Autodesk Fusion 360 part; units mm, degrees
(part 5 of 10)
  line L3608 (-26.7971, 36.5251) -> (-27.0734, 36.4711)
  line L3609 (-27.0734, 36.4711) -> (-27.3544, 36.4533)
  line L3610 (-27.3544, 36.4533) -> (-27.6353, 36.4722)
  line L3611 (-27.6353, 36.4722) -> (-27.9114, 36.5273)
  line L3612 (-27.9114, 36.5273) -> (-28.1781, 36.6178)
  line L3613 (-28.1781, 36.6178) -> (-28.4307, 36.7421)
  line L3614 (-28.4307, 36.7421) -> (-28.6651, 36.8981)
  line L3615 (-28.6651, 36.8981) -> (-28.8773, 37.0832)
  line L3616 (-28.8773, 37.0832) -> (-29.0637, 37.2942)
  line L3617 (-29.0637, 37.2942) -> (-29.2211, 37.5276)
  line L3618 (-29.2211, 37.5276) -> (-29.347, 37.7794)
  line L3619 (-29.347, 37.7794) -> (-29.4391, 38.0455)
  line L3620 (-29.4391, 38.0455) -> (-29.496, 38.3212)
  line L3621 (-29.496, 38.3212) -> (-29.5166, 38.602)
  line L3622 (-29.5166, 38.602) -> (-29.5006, 38.8831)
  line L3623 (-29.5006, 38.8831) -> (-29.4484, 39.1598)
  line L3624 (-29.4484, 39.1598) -> (-29.3606, 39.4273)
  line L3625 (-29.3606, 39.4273) -> (-29.3282, 39.495)
  line L3626 (-29.3282, 39.495) -> (-30.1357, 39.495)
  line L3627 (-30.1357, 39.495) -> (-30.1651, 39.411)
  line L3628 (-30.1651, 39.411) -> (-30.2382, 39.0907)
  line L3629 (-30.2382, 39.0907) -> (-30.275, 38.7643)
  line L3630 (-30.275, 38.7643) -> (-30.275, 38.4357)
  line L3631 (-26.8401, 42.0374) -> (-26.5056, 41.9709)
  line L3632 (-26.5056, 41.9709) -> (-26.1793, 41.8719)
  line L3633 (-26.1793, 41.8719) -> (-25.8642, 41.7414)
  line L3634 (-25.8642, 41.7414) -> (-25.5635, 41.5806)
  line L3635 (-25.5635, 41.5806) -> (-25.2799, 41.3911)
  line L3636 (-25.2799, 41.3911) -> (-25.0163, 41.1748)
  line L3637 (-25.0163, 41.1748) -> (-24.7752, 40.9337)
  line L3638 (-24.7752, 40.9337) -> (-24.5589, 40.6701)
  line L3639 (-24.5589, 40.6701) -> (-24.3694, 40.3865)
  line L3640 (-24.3694, 40.3865) -> (-24.2086, 40.0858)
  line L3641 (-24.2086, 40.0858) -> (-24.0781, 39.7707)
  line L3642 (-24.0781, 39.7707) -> (-23.9791, 39.4444)
  line L3643 (-23.9791, 39.4444) -> (-23.9126, 39.1099)
  line L3644 (-23.9126, 39.1099) -> (-23.8792, 38.7705)
  line L3645 (-23.8792, 38.7705) -> (-23.8792, 38.4295)
  line L3646 (-23.8792, 38.4295) -> (-23.9126, 38.0901)
  line L3647 (-23.9126, 38.0901) -> (-23.9791, 37.7556)
  line L3648 (-23.9791, 37.7556) -> (-24.0781, 37.4293)
  line L3649 (-24.0781, 37.4293) -> (-24.2086, 37.1142)
  line L3650 (-24.2086, 37.1142) -> (-24.3694, 36.8135)
  line L3651 (-24.3694, 36.8135) -> (-24.5589, 36.5299)
  line L3652 (-24.5589, 36.5299) -> (-24.7752, 36.2663)
  line L3653 (-24.7752, 36.2663) -> (-25.0163, 36.0252)
  line L3654 (-25.0163, 36.0252) -> (-25.2799, 35.8089)
  line L3655 (-25.2799, 35.8089) -> (-25.5635, 35.6194)
  line L3656 (-25.5635, 35.6194) -> (-25.8642, 35.4586)
  line L3657 (-25.8642, 35.4586) -> (-26.1793, 35.3281)
  line L3658 (-26.1793, 35.3281) -> (-26.5056, 35.2291)
  line L3659 (-26.5056, 35.2291) -> (-26.8401, 35.1626)
  line L3660 (-26.8401, 35.1626) -> (-27.1795, 35.1292)
  line L3661 (-27.1795, 35.1292) -> (-27.5205, 35.1292)
  line L3662 (-27.5205, 35.1292) -> (-27.8599, 35.1626)
  line L3663 (-27.8599, 35.1626) -> (-28.1944, 35.2291)
  line L3664 (-28.1944, 35.2291) -> (-28.5207, 35.3281)
  line L3665 (-28.5207, 35.3281) -> (-28.8358, 35.4586)
  line L3666 (-28.8358, 35.4586) -> (-29.1365, 35.6194)
  line L3667 (-29.1365, 35.6194) -> (-29.4201, 35.8089)
  line L3668 (-29.4201, 35.8089) -> (-29.6837, 36.0252)
  line L3669 (-29.6837, 36.0252) -> (-29.9248, 36.2663)
  line L3670 (-29.9248, 36.2663) -> (-30.1411, 36.5299)
  line L3671 (-30.1411, 36.5299) -> (-30.3306, 36.8135)
  line L3672 (-30.3306, 36.8135) -> (-30.4914, 37.1142)
  line L3673 (-30.4914, 37.1142) -> (-30.6219, 37.4293)
  line L3674 (-30.6219, 37.4293) -> (-30.7209, 37.7556)
  line L3675 (-30.7209, 37.7556) -> (-30.7874, 38.0901)
  line L3676 (-30.7874, 38.0901) -> (-30.8208, 38.4295)
  line L3677 (-30.8208, 38.4295) -> (-30.8208, 38.7705)
  line L3678 (-30.8208, 38.7705) -> (-30.8198, 38.7811)
  line L3679 (-30.8198, 38.7811) -> (-30.7874, 39.1099)
  line L3680 (-30.7874, 39.1099) -> (-30.7209, 39.4444)
  line L3681 (-30.7209, 39.4444) -> (-30.6219, 39.7707)
  line L3682 (-30.6219, 39.7707) -> (-30.4914, 40.0858)
  line L3683 (-30.4914, 40.0858) -> (-30.3306, 40.3865)
  line L3684 (-30.3306, 40.3865) -> (-30.1411, 40.6701)
  line L3685 (-30.1411, 40.6701) -> (-29.9248, 40.9337)
  line L3686 (-29.9248, 40.9337) -> (-29.6837, 41.1748)
  line L3687 (-29.6837, 41.1748) -> (-29.4201, 41.3911)
  line L3688 (-29.4201, 41.3911) -> (-29.1365, 41.5806)
  line L3689 (-29.1365, 41.5806) -> (-28.8358, 41.7414)
  line L3690 (-28.8358, 41.7414) -> (-28.5207, 41.8719)
  line L3691 (-28.5207, 41.8719) -> (-28.1944, 41.9709)
  line L3692 (-28.1944, 41.9709) -> (-27.8599, 42.0374)
  line L3693 (-27.8599, 42.0374) -> (-27.5205, 42.0708)
  line L3694 (-27.5205, 42.0708) -> (-27.1795, 42.0708)
  line L3695 (-27.1795, 42.0708) -> (-26.8401, 42.0374)
  line L3696 (-30.575, 38.4189) -> (-30.5344, 38.0589)
  line L3697 (-30.5344, 38.0589) -> (-30.4538, 37.7058)
  line L3698 (-30.4538, 37.7058) -> (-30.3342, 37.3639)
  line L3699 (-30.3342, 37.3639) -> (-30.177, 37.0375)
  line L3700 (-30.177, 37.0375) -> (-29.9843, 36.7308)
  line L3701 (-29.9843, 36.7308) -> (-29.7585, 36.4476)
  line L3702 (-29.7585, 36.4476) -> (-29.5024, 36.1915)
  line L3703 (-29.5024, 36.1915) -> (-29.2192, 35.9657)
  line L3704 (-29.2192, 35.9657) -> (-28.9125, 35.773)
  line L3705 (-28.9125, 35.773) -> (-28.5861, 35.6158)
  line L3706 (-28.5861, 35.6158) -> (-28.2442, 35.4962)
  line L3707 (-28.2442, 35.4962) -> (-27.8911, 35.4156)
  line L3708 (-27.8911, 35.4156) -> (-27.5311, 35.375)
  line L3709 (-27.5311, 35.375) -> (-27.1689, 35.375)
  line L3710 (-27.1689, 35.375) -> (-26.8089, 35.4156)
  line L3711 (-26.8089, 35.4156) -> (-26.4558, 35.4962)
  line L3712 (-26.4558, 35.4962) -> (-26.1139, 35.6158)
  line L3713 (-26.1139, 35.6158) -> (-25.7875, 35.773)
  line L3714 (-25.7875, 35.773) -> (-25.4808, 35.9657)
  line L3715 (-25.4808, 35.9657) -> (-25.1976, 36.1915)
  line L3716 (-25.1976, 36.1915) -> (-24.9415, 36.4476)
  line L3717 (-24.9415, 36.4476) -> (-24.7157, 36.7308)
  line L3718 (-24.7157, 36.7308) -> (-24.523, 37.0375)
  line L3719 (-24.523, 37.0375) -> (-24.3658, 37.3639)
  line L3720 (-24.3658, 37.3639) -> (-24.2462, 37.7058)
  line L3721 (-24.2462, 37.7058) -> (-24.1656, 38.0589)
  line L3722 (-24.1656, 38.0589) -> (-24.125, 38.4189)
  line L3723 (-24.125, 38.4189) -> (-24.125, 38.7811)
  line L3724 (-24.125, 38.7811) -> (-24.1656, 39.1411)
  line L3725 (-24.1656, 39.1411) -> (-24.2462, 39.4942)
  line L3726 (-24.2462, 39.4942) -> (-24.3658, 39.8361)
  line L3727 (-24.3658, 39.8361) -> (-24.523, 40.1625)
  line L3728 (-24.523, 40.1625) -> (-24.7157, 40.4692)
  line L3729 (-24.7157, 40.4692) -> (-24.9415, 40.7524)
  line L3730 (-24.9415, 40.7524) -> (-25.1976, 41.0085)
  line L3731 (-25.1976, 41.0085) -> (-25.4808, 41.2343)
  line L3732 (-25.4808, 41.2343) -> (-25.7875, 41.427)
  line L3733 (-25.7875, 41.427) -> (-26.1139, 41.5842)
  line L3734 (-26.1139, 41.5842) -> (-26.4558, 41.7038)
  line L3735 (-26.4558, 41.7038) -> (-26.8089, 41.7844)
  line L3736 (-26.8089, 41.7844) -> (-27.1689, 41.825)
  line L3737 (-27.1689, 41.825) -> (-27.5311, 41.825)
  line L3738 (-27.5311, 41.825) -> (-27.8911, 41.7844)
  line L3739 (-27.8911, 41.7844) -> (-28.2442, 41.7038)
  line L3740 (-28.2442, 41.7038) -> (-28.5861, 41.5842)
  line L3741 (-28.5861, 41.5842) -> (-28.9125, 41.427)
  line L3742 (-28.9125, 41.427) -> (-29.2192, 41.2343)
  line L3743 (-29.2192, 41.2343) -> (-29.5024, 41.0085)
  line L3744 (-29.5024, 41.0085) -> (-29.7585, 40.7524)
  line L3745 (-29.7585, 40.7524) -> (-29.9843, 40.4692)
  line L3746 (-29.9843, 40.4692) -> (-30.177, 40.1625)
  line L3747 (-30.177, 40.1625) -> (-30.3342, 39.8361)
  line L3748 (-30.3342, 39.8361) -> (-30.4538, 39.4942)
  line L3749 (-30.4538, 39.4942) -> (-30.5344, 39.1411)
  line L3750 (-30.5344, 39.1411) -> (-30.575, 38.7811)
  line L3751 (-30.575, 38.7811) -> (-30.575, 38.4189)
  line L3752 (-26.7535, 42.621) -> (-26.3623, 42.5432)
  line L3753 (-26.3623, 42.5432) -> (-25.9805, 42.4274)
  line L3754 (-25.9805, 42.4274) -> (-25.612, 42.2747)
  line L3755 (-25.612, 42.2747) -> (-25.2602, 42.0867)
  line L3756 (-25.2602, 42.0867) -> (-24.9285, 41.865)
  line L3757 (-24.9285, 41.865) -> (-24.6201, 41.612)
  line L3758 (-24.6201, 41.612) -> (-24.338, 41.3299)
  line L3759 (-24.338, 41.3299) -> (-24.085, 41.0215)
  line L3760 (-24.085, 41.0215) -> (-23.8633, 40.6898)
  line L3761 (-23.8633, 40.6898) -> (-23.6753, 40.338)
  line L3762 (-23.6753, 40.338) -> (-23.5226, 39.9695)
  line L3763 (-23.5226, 39.9695) -> (-23.4068, 39.5877)
  line L3764 (-23.4068, 39.5877) -> (-23.329, 39.1965)
  line L3765 (-23.329, 39.1965) -> (-23.2899, 38.7995)
  line L3766 (-23.2899, 38.7995) -> (-23.2899, 38.4005)
  line L3767 (-23.2899, 38.4005) -> (-23.329, 38.0035)
  line L3768 (-23.329, 38.0035) -> (-23.4068, 37.6123)
  line L3769 (-23.4068, 37.6123) -> (-23.5226, 37.2305)
  line L3770 (-23.5226, 37.2305) -> (-23.6753, 36.862)
  line L3771 (-23.6753, 36.862) -> (-23.8633, 36.5102)
  line L3772 (-23.8633, 36.5102) -> (-24.085, 36.1785)
  line L3773 (-24.085, 36.1785) -> (-24.338, 35.8701)
  line L3774 (-24.338, 35.8701) -> (-24.6201, 35.588)
  line L3775 (-24.6201, 35.588) -> (-24.9285, 35.335)
  line L3776 (-24.9285, 35.335) -> (-25.2602, 35.1133)
  line L3777 (-25.2602, 35.1133) -> (-25.612, 34.9253)
  line L3778 (-25.612, 34.9253) -> (-25.9805, 34.7726)
  line L3779 (-25.9805, 34.7726) -> (-26.3623, 34.6568)
  line L3780 (-26.3623, 34.6568) -> (-26.7535, 34.579)
  line L3781 (-26.7535, 34.579) -> (-27.1505, 34.5399)
  line L3782 (-27.1505, 34.5399) -> (-27.5495, 34.5399)
  line L3783 (-27.5495, 34.5399) -> (-27.9465, 34.579)
  line L3784 (-27.9465, 34.579) -> (-28.3377, 34.6568)
  line L3785 (-28.3377, 34.6568) -> (-28.7195, 34.7726)
  line L3786 (-28.7195, 34.7726) -> (-29.088, 34.9253)
  line L3787 (-29.088, 34.9253) -> (-29.4398, 35.1133)
  line L3788 (-29.4398, 35.1133) -> (-29.7715, 35.335)
  line L3789 (-29.7715, 35.335) -> (-30.0799, 35.588)
  line L3790 (-30.0799, 35.588) -> (-30.362, 35.8701)
  line L3791 (-30.362, 35.8701) -> (-30.615, 36.1785)
  line L3792 (-30.615, 36.1785) -> (-30.8367, 36.5102)
  line L3793 (-30.8367, 36.5102) -> (-31.0247, 36.862)
  line L3794 (-31.0247, 36.862) -> (-31.1774, 37.2305)
  line L3795 (-31.1774, 37.2305) -> (-31.2932, 37.6123)
  line L3796 (-31.2932, 37.6123) -> (-31.371, 38.0035)
  line L3797 (-31.371, 38.0035) -> (-31.4101, 38.4005)
  line L3798 (-31.4101, 38.4005) -> (-31.4101, 38.7874)
  line L3799 (-31.4101, 38.7874) -> (-31.4101, 38.7995)
  line L3800 (-31.4101, 38.7995) -> (-31.371, 39.1965)
  line L3801 (-31.371, 39.1965) -> (-31.2932, 39.5877)
  line L3802 (-31.2932, 39.5877) -> (-31.1774, 39.9695)
  line L3803 (-31.1774, 39.9695) -> (-31.0247, 40.338)
  line L3804 (-31.0247, 40.338) -> (-30.8367, 40.6898)
  line L3805 (-30.8367, 40.6898) -> (-30.615, 41.0215)
  line L3806 (-30.615, 41.0215) -> (-30.362, 41.3299)
  line L3807 (-30.362, 41.3299) -> (-30.0799, 41.612)
  line L3808 (-30.0799, 41.612) -> (-29.7715, 41.865)
  line L3809 (-29.7715, 41.865) -> (-29.4398, 42.0867)
  line L3810 (-29.4398, 42.0867) -> (-29.088, 42.2747)
  line L3811 (-29.088, 42.2747) -> (-28.7195, 42.4274)
  line L3812 (-28.7195, 42.4274) -> (-28.3377, 42.5432)
  line L3813 (-28.3377, 42.5432) -> (-27.9465, 42.621)
  line L3814 (-27.9465, 42.621) -> (-27.5495, 42.6601)
  line L3815 (-27.5495, 42.6601) -> (-27.1505, 42.6601)
  line L3816 (-27.1505, 42.6601) -> (-26.7535, 42.621)
  line L3817 (-31.165, 38.4126) -> (-31.1283, 38.0395)
  line L3818 (-31.1283, 38.0395) -> (-31.0551, 37.6719)
  line L3819 (-31.0551, 37.6719) -> (-30.9463, 37.3132)
  line L3820 (-30.9463, 37.3132) -> (-30.8029, 36.9669)
  line L3821 (-30.8029, 36.9669) -> (-30.6262, 36.6363)
  line L3822 (-30.6262, 36.6363) -> (-30.4179, 36.3247)
  line L3823 (-30.4179, 36.3247) -> (-30.1801, 36.0349)
  line L3824 (-30.1801, 36.0349) -> (-29.9151, 35.7699)
  line L3825 (-29.9151, 35.7699) -> (-29.6253, 35.5321)
  line L3826 (-29.6253, 35.5321) -> (-29.3137, 35.3238)
  line L3827 (-29.3137, 35.3238) -> (-28.9831, 35.1471)
  line L3828 (-28.9831, 35.1471) -> (-28.6368, 35.0037)
  line L3829 (-28.6368, 35.0037) -> (-28.2781, 34.8949)
  line L3830 (-28.2781, 34.8949) -> (-27.9105, 34.8217)
  line L3831 (-27.9105, 34.8217) -> (-27.5374, 34.785)
  line L3832 (-27.5374, 34.785) -> (-27.1626, 34.785)
  line L3833 (-27.1626, 34.785) -> (-26.7895, 34.8217)
  line L3834 (-26.7895, 34.8217) -> (-26.4219, 34.8949)
  line L3835 (-26.4219, 34.8949) -> (-26.0632, 35.0037)
  line L3836 (-26.0632, 35.0037) -> (-25.7169, 35.1471)
  line L3837 (-25.7169, 35.1471) -> (-25.3863, 35.3238)
  line L3838 (-25.3863, 35.3238) -> (-25.0747, 35.5321)
  line L3839 (-25.0747, 35.5321) -> (-24.7849, 35.7699)
  line L3840 (-24.7849, 35.7699) -> (-24.5199, 36.0349)
  line L3841 (-24.5199, 36.0349) -> (-24.2821, 36.3247)
  line L3842 (-24.2821, 36.3247) -> (-24.0738, 36.6363)
  line L3843 (-24.0738, 36.6363) -> (-23.8971, 36.9669)
  line L3844 (-23.8971, 36.9669) -> (-23.7537, 37.3132)
  line L3845 (-23.7537, 37.3132) -> (-23.6449, 37.6719)
  line L3846 (-23.6449, 37.6719) -> (-23.5717, 38.0395)
  line L3847 (-23.5717, 38.0395) -> (-23.535, 38.4126)
  line L3848 (-23.535, 38.4126) -> (-23.535, 38.7874)
  line L3849 (-23.535, 38.7874) -> (-23.5717, 39.1605)
  line L3850 (-23.5717, 39.1605) -> (-23.6449, 39.5281)
  line L3851 (-23.6449, 39.5281) -> (-23.7537, 39.8868)
  line L3852 (-23.7537, 39.8868) -> (-23.8971, 40.2331)
  line L3853 (-23.8971, 40.2331) -> (-24.0738, 40.5637)
  line L3854 (-24.0738, 40.5637) -> (-24.2821, 40.8753)
  line L3855 (-24.2821, 40.8753) -> (-24.5199, 41.1651)
  line L3856 (-24.5199, 41.1651) -> (-24.7849, 41.4301)
  line L3857 (-24.7849, 41.4301) -> (-25.0747, 41.6679)
  line L3858 (-25.0747, 41.6679) -> (-25.3863, 41.8762)
  line L3859 (-25.3863, 41.8762) -> (-25.7169, 42.0529)
  line L3860 (-25.7169, 42.0529) -> (-26.0632, 42.1963)
  line L3861 (-26.0632, 42.1963) -> (-26.4219, 42.3051)
  line L3862 (-26.4219, 42.3051) -> (-26.7895, 42.3783)
  line L3863 (-26.7895, 42.3783) -> (-27.1626, 42.415)
  line L3864 (-27.1626, 42.415) -> (-27.5374, 42.415)
  line L3865 (-27.5374, 42.415) -> (-27.9105, 42.3783)
  line L3866 (-27.9105, 42.3783) -> (-28.2781, 42.3051)
  line L3867 (-28.2781, 42.3051) -> (-28.6368, 42.1963)
  line L3868 (-28.6368, 42.1963) -> (-28.9831, 42.0529)
  line L3869 (-28.9831, 42.0529) -> (-29.3137, 41.8762)
  line L3870 (-29.3137, 41.8762) -> (-29.6253, 41.6679)
  line L3871 (-29.6253, 41.6679) -> (-29.9151, 41.4301)
  line L3872 (-29.9151, 41.4301) -> (-30.1801, 41.1651)
  line L3873 (-30.1801, 41.1651) -> (-30.4179, 40.8753)
  line L3874 (-30.4179, 40.8753) -> (-30.6262, 40.5637)
  line L3875 (-30.6262, 40.5637) -> (-30.8029, 40.2331)
  line L3876 (-30.8029, 40.2331) -> (-30.9463, 39.8868)
  line L3877 (-30.9463, 39.8868) -> (-31.0551, 39.5281)
  line L3878 (-31.0551, 39.5281) -> (-31.1283, 39.1605)
  line L3879 (-31.1283, 39.1605) -> (-31.165, 38.7874)
  line L3880 (-31.165, 38.7874) -> (-31.165, 38.4126)
  line L3881 (-30.3956, 44.7226) -> (-30.3506, 44.7039)
  line L3882 (-30.3506, 44.7039) -> (-30.3161, 44.6694)
  line L3883 (-30.3161, 44.6694) -> (-30.2974, 44.6244)
  line L3884 (-30.2974, 44.6244) -> (-30.2974, 44.5756)
  line L3885 (-30.2974, 44.5756) -> (-30.3161, 44.5306)
  line L3886 (-30.3161, 44.5306) -> (-30.3506, 44.4961)
  line L3887 (-30.3506, 44.4961) -> (-30.3956, 44.4774)
  line L3888 (-30.3956, 44.4774) -> (-30.42, 44.475)
  line L3889 (-30.42, 44.475) -> (-33.04, 44.475)
  line L3890 (-33.04, 44.475) -> (-33.0644, 44.4774)
  line L3891 (-33.0644, 44.4774) -> (-33.1094, 44.4961)
  line L3892 (-33.1094, 44.4961) -> (-33.125, 44.5116)
  line L3893 (-33.125, 44.5116) -> (-33.125, 40.77)
  line L3894 (-33.125, 40.77) -> (-33.1274, 40.7456)
  line L3895 (-33.1274, 40.7456) -> (-33.1461, 40.7006)
  line L3896 (-33.1461, 40.7006) -> (-33.1806, 40.6661)
  line L3897 (-33.1806, 40.6661) -> (-33.2256, 40.6474)
  line L3898 (-33.2256, 40.6474) -> (-33.2744, 40.6474)
  line L3899 (-33.2744, 40.6474) -> (-33.3194, 40.6661)
  line L3900 (-33.3194, 40.6661) -> (-33.3539, 40.7006)
  line L3901 (-33.3539, 40.7006) -> (-33.3726, 40.7456)
  line L3902 (-33.3726, 40.7456) -> (-33.375, 40.77)
  line L3903 (-33.375, 40.77) -> (-33.375, 44.6)
  line L3904 (-33.375, 44.6) -> (-33.3726, 44.6244)
  line L3905 (-33.3726, 44.6244) -> (-33.3539, 44.6694)
  line L3906 (-33.3539, 44.6694) -> (-33.3194, 44.7039)
  line L3907 (-33.3194, 44.7039) -> (-33.2744, 44.7226)
  line L3908 (-33.2744, 44.7226) -> (-33.2256, 44.7226)
  line L3909 (-33.2256, 44.7226) -> (-33.1806, 44.7039)
  line L3910 (-33.1806, 44.7039) -> (-33.1461, 44.6694)
  line L3911 (-33.1461, 44.6694) -> (-33.145, 44.6669)
  line L3912 (-33.145, 44.6669) -> (-33.1439, 44.6694)
  line L3913 (-33.1439, 44.6694) -> (-33.1094, 44.7039)
  line L3914 (-33.1094, 44.7039) -> (-33.0644, 44.7226)
  line L3915 (-33.0644, 44.7226) -> (-33.04, 44.725)
  line L3916 (-33.04, 44.725) -> (-30.42, 44.725)
  line L3917 (-30.42, 44.725) -> (-30.3956, 44.7226)
  line L3918 (-21.4256, 44.7226) -> (-21.3806, 44.7039)
  line L3919 (-21.3806, 44.7039) -> (-21.3461, 44.6694)
  line L3920 (-21.3461, 44.6694) -> (-21.3274, 44.6244)
  line L3921 (-21.3274, 44.6244) -> (-21.325, 44.6)
  line L3922 (-21.325, 44.6) -> (-21.325, 40.77)
  line L3923 (-21.325, 40.77) -> (-21.3274, 40.7456)
  line L3924 (-21.3274, 40.7456) -> (-21.3461, 40.7006)
  line L3925 (-21.3461, 40.7006) -> (-21.3806, 40.6661)
  line L3926 (-21.3806, 40.6661) -> (-21.4256, 40.6474)
  line L3927 (-21.4256, 40.6474) -> (-21.4744, 40.6474)
  line L3928 (-21.4744, 40.6474) -> (-21.5194, 40.6661)
  line L3929 (-21.5194, 40.6661) -> (-21.5539, 40.7006)
  line L3930 (-21.5539, 40.7006) -> (-21.5726, 40.7456)
  line L3931 (-21.5726, 40.7456) -> (-21.575, 40.77)
  line L3932 (-21.575, 40.77) -> (-21.575, 44.475)
  line L3933 (-21.575, 44.475) -> (-24.28, 44.475)
  line L3934 (-24.28, 44.475) -> (-24.3044, 44.4774)
  line L3935 (-24.3044, 44.4774) -> (-24.3494, 44.4961)
  line L3936 (-24.3494, 44.4961) -> (-24.3839, 44.5306)
  line L3937 (-24.3839, 44.5306) -> (-24.4026, 44.5756)
  line L3938 (-24.4026, 44.5756) -> (-24.4026, 44.6244)
  line L3939 (-24.4026, 44.6244) -> (-24.3839, 44.6694)
  line L3940 (-24.3839, 44.6694) -> (-24.3494, 44.7039)
  line L3941 (-24.3494, 44.7039) -> (-24.3044, 44.7226)
  line L3942 (-24.3044, 44.7226) -> (-24.28, 44.725)
  line L3943 (-24.28, 44.725) -> (-21.45, 44.725)
  line L3944 (-21.45, 44.725) -> (-21.4256, 44.7226)
  line L3945 (-25.3156, 44.7226) -> (-25.2706, 44.7039)
  line L3946 (-25.2706, 44.7039) -> (-25.2361, 44.6694)
  line L3947 (-25.2361, 44.6694) -> (-25.2174, 44.6244)
  line L3948 (-25.2174, 44.6244) -> (-25.2174, 44.5756)
  line L3949 (-25.2174, 44.5756) -> (-25.2361, 44.5306)
  line L3950 (-25.2361, 44.5306) -> (-25.2706, 44.4961)
  line L3951 (-25.2706, 44.4961) -> (-25.3156, 44.4774)
  line L3952 (-25.3156, 44.4774) -> (-25.34, 44.475)
  line L3953 (-25.34, 44.475) -> (-29.36, 44.475)
  line L3954 (-29.36, 44.475) -> (-29.3844, 44.4774)
  line L3955 (-29.3844, 44.4774) -> (-29.4294, 44.4961)
  line L3956 (-29.4294, 44.4961) -> (-29.4639, 44.5306)
  line L3957 (-29.4639, 44.5306) -> (-29.4826, 44.5756)
  line L3958 (-29.4826, 44.5756) -> (-29.4826, 44.6244)
  line L3959 (-29.4826, 44.6244) -> (-29.4639, 44.6694)
  line L3960 (-29.4639, 44.6694) -> (-29.4294, 44.7039)
  line L3961 (-29.4294, 44.7039) -> (-29.3844, 44.7226)
  line L3962 (-29.3844, 44.7226) -> (-29.36, 44.725)
  line L3963 (-29.36, 44.725) -> (-25.34, 44.725)
  line L3964 (-25.34, 44.725) -> (-25.3156, 44.7226)
  line L3965 (-21.4446, 45.773) -> (-21.4446, 45.727)
  line L3966 (-21.4446, 45.727) -> (-21.477, 45.6946)
  line L3967 (-21.477, 45.6946) -> (-21.523, 45.6946)
  line L3968 (-21.523, 45.6946) -> (-21.5554, 45.727)
  line L3969 (-21.5554, 45.727) -> (-21.5554, 45.773)
  line L3970 (-21.5554, 45.773) -> (-21.523, 45.8054)
  line L3971 (-21.523, 45.8054) -> (-21.477, 45.8054)
  line L3972 (-21.477, 45.8054) -> (-21.4446, 45.773)
  line L3973 (-15.9694, 47.7992) -> (-15.8993, 47.7291)
  line L3974 (-15.8993, 47.7291) -> (-15.8614, 47.6375)
  line L3975 (-15.8614, 47.6375) -> (-15.8614, 47.5384)
  line L3976 (-15.8614, 47.5384) -> (-15.8993, 47.4469)
  line L3977 (-15.8993, 47.4469) -> (-15.9694, 47.3768)
  line L3978 (-15.9694, 47.3768) -> (-16.0609, 47.3389)
  line L3979 (-16.0609, 47.3389) -> (-16.1601, 47.3389)
  line L3980 (-16.1601, 47.3389) -> (-16.2516, 47.3768)
  line L3981 (-16.2516, 47.3768) -> (-16.3217, 47.4469)
  line L3982 (-16.3217, 47.4469) -> (-16.3596, 47.5384)
  line L3983 (-16.3596, 47.5384) -> (-16.3596, 47.6375)
  line L3984 (-16.3596, 47.6375) -> (-16.3217, 47.7291)
  line L3985 (-16.3217, 47.7291) -> (-16.2516, 47.7992)
  line L3986 (-16.2516, 47.7992) -> (-16.1601, 47.8371)
  line L3987 (-16.1601, 47.8371) -> (-16.0609, 47.8371)
  line L3988 (-16.0609, 47.8371) -> (-15.9694, 47.7992)
  line L3989 (-27.5973, 48.6187) -> (-27.5948, 48.6177)
  line L3990 (-27.5948, 48.6177) -> (-27.5921, 48.6175)
  line L3991 (-27.5921, 48.6175) -> (-27.5784, 48.6123)
  line L3992 (-27.5784, 48.6123) -> (-27.4831, 48.5646)
  line L3993 (-27.4831, 48.5646) -> (-27.4768, 48.5607)
  line L3994 (-27.4768, 48.5607) -> (-27.475, 48.5599)
  line L3995 (-27.475, 48.5599) -> (-27.4729, 48.5582)
  line L3996 (-27.4729, 48.5582) -> (-27.4707, 48.5568)
  line L3997 (-27.4707, 48.5568) -> (-27.4694, 48.5553)
  line L3998 (-27.4694, 48.5553) -> (-27.4636, 48.5506)
  line L3999 (-27.4636, 48.5506) -> (-27.3684, 48.4554)
  line L4000 (-27.3684, 48.4554) -> (-27.3591, 48.444)
  line L4001 (-27.3591, 48.444) -> (-27.3569, 48.4388)
  line L4002 (-27.3569, 48.4388) -> (-27.3536, 48.4344)
  line L4003 (-27.3536, 48.4344) -> (-27.3487, 48.4205)
  line L4004 (-27.3487, 48.4205) -> (-27.301, 48.23)
  line L4005 (-27.301, 48.23) -> (-27.3007, 48.2275)
  line L4006 (-27.3007, 48.2275) -> (-27.3003, 48.2265)
  line L4007 (-27.3003, 48.2265) -> (-27.2997, 48.221)
  line L4008 (-27.2997, 48.221) -> (-27.2989, 48.2155)
  line L4009 (-27.2989, 48.2155) -> (-27.2991, 48.2144)
  line L4010 (-27.2991, 48.2144) -> (-27.2988, 48.2118)
  line L4011 (-27.2988, 48.2118) -> (-27.2988, 47.8785)
  line L4012 (-27.2988, 47.8785) -> (-27.2991, 47.876)
  line L4013 (-27.2991, 47.876) -> (-27.2989, 47.8749)
  line L4014 (-27.2989, 47.8749) -> (-27.2997, 47.8694)
  line L4015 (-27.2997, 47.8694) -> (-27.3003, 47.8639)
  line L4016 (-27.3003, 47.8639) -> (-27.3007, 47.8629)
  line L4017 (-27.3007, 47.8629) -> (-27.301, 47.8603)
  line L4018 (-27.301, 47.8603) -> (-27.3487, 47.6698)
  line L4019 (-27.3487, 47.6698) -> (-27.3536, 47.656)
  line L4020 (-27.3536, 47.656) -> (-27.3569, 47.6515)
  line L4021 (-27.3569, 47.6515) -> (-27.3591, 47.6464)
  line L4022 (-27.3591, 47.6464) -> (-27.3684, 47.635)
  line L4023 (-27.3684, 47.635) -> (-27.4636, 47.5398)
  line L4024 (-27.4636, 47.5398) -> (-27.4694, 47.535)
  line L4025 (-27.4694, 47.535) -> (-27.4707, 47.5335)
  line L4026 (-27.4707, 47.5335) -> (-27.4729, 47.5321)
  line L4027 (-27.4729, 47.5321) -> (-27.475, 47.5304)
  line L4028 (-27.475, 47.5304) -> (-27.4768, 47.5297)
  line L4029 (-27.4768, 47.5297) -> (-27.4831, 47.5257)
  line L4030 (-27.4831, 47.5257) -> (-27.5784, 47.4781)
  line L4031 (-27.5784, 47.4781) -> (-27.5921, 47.4728)
  line L4032 (-27.5921, 47.4728) -> (-27.5948, 47.4727)
  line L4033 (-27.5948, 47.4727) -> (-27.5973, 47.4716)
  line L4034 (-27.5973, 47.4716) -> (-27.6119, 47.4702)
  line L4035 (-27.6119, 47.4702) -> (-27.8024, 47.4702)
  line L4036 (-27.8024, 47.4702) -> (-27.817, 47.4716)
  line L4037 (-27.817, 47.4716) -> (-27.8195, 47.4727)
  line L4038 (-27.8195, 47.4727) -> (-27.8222, 47.4728)
  line L4039 (-27.8222, 47.4728) -> (-27.8359, 47.4781)
  line L4040 (-27.8359, 47.4781) -> (-27.9312, 47.5257)
  line L4041 (-27.9312, 47.5257) -> (-27.9375, 47.5297)
  line L4042 (-27.9375, 47.5297) -> (-27.9393, 47.5304)
  line L4043 (-27.9393, 47.5304) -> (-27.9413, 47.5321)
  line L4044 (-27.9413, 47.5321) -> (-27.9436, 47.5335)
  line L4045 (-27.9436, 47.5335) -> (-27.9449, 47.535)
  line L4046 (-27.9449, 47.535) -> (-27.9507, 47.5398)
  line L4047 (-27.9507, 47.5398) -> (-28.0459, 47.635)
  line L4048 (-28.0459, 47.635) -> (-28.0552, 47.6464)
  line L4049 (-28.0552, 47.6464) -> (-28.0574, 47.6515)
  line L4050 (-28.0574, 47.6515) -> (-28.0607, 47.656)
  line L4051 (-28.0607, 47.656) -> (-28.0656, 47.6698)
  line L4052 (-28.0656, 47.6698) -> (-28.1132, 47.8603)
  line L4053 (-28.1132, 47.8603) -> (-28.1136, 47.8629)
  line L4054 (-28.1136, 47.8629) -> (-28.114, 47.8639)
  line L4055 (-28.114, 47.8639) -> (-28.1146, 47.8694)
  line L4056 (-28.1146, 47.8694) -> (-28.1154, 47.8749)
  line L4057 (-28.1154, 47.8749) -> (-28.1152, 47.876)
  line L4058 (-28.1152, 47.876) -> (-28.1155, 47.8785)
  line L4059 (-28.1155, 47.8785) -> (-28.1155, 48.2118)
  line L4060 (-28.1155, 48.2118) -> (-28.1152, 48.2144)
  line L4061 (-28.1152, 48.2144) -> (-28.1154, 48.2155)
  line L4062 (-28.1154, 48.2155) -> (-28.1146, 48.221)
  line L4063 (-28.1146, 48.221) -> (-28.114, 48.2265)
  line L4064 (-28.114, 48.2265) -> (-28.1136, 48.2275)
  line L4065 (-28.1136, 48.2275) -> (-28.1132, 48.23)
  line L4066 (-28.1132, 48.23) -> (-28.0656, 48.4205)
  line L4067 (-28.0656, 48.4205) -> (-28.0607, 48.4344)
  line L4068 (-28.0607, 48.4344) -> (-28.0574, 48.4388)
  line L4069 (-28.0574, 48.4388) -> (-28.0552, 48.444)
  line L4070 (-28.0552, 48.444) -> (-28.0459, 48.4554)
  line L4071 (-28.0459, 48.4554) -> (-27.9507, 48.5506)
  line L4072 (-27.9507, 48.5506) -> (-27.9449, 48.5553)
  line L4073 (-27.9449, 48.5553) -> (-27.9436, 48.5568)
  line L4074 (-27.9436, 48.5568) -> (-27.9413, 48.5582)
  line L4075 (-27.9413, 48.5582) -> (-27.9393, 48.5599)
  line L4076 (-27.9393, 48.5599) -> (-27.9375, 48.5607)
  line L4077 (-27.9375, 48.5607) -> (-27.9312, 48.5646)
  line L4078 (-27.9312, 48.5646) -> (-27.8359, 48.6123)
  line L4079 (-27.8359, 48.6123) -> (-27.8222, 48.6175)
  line L4080 (-27.8222, 48.6175) -> (-27.8195, 48.6177)
  line L4081 (-27.8195, 48.6177) -> (-27.817, 48.6187)
  line L4082 (-27.817, 48.6187) -> (-27.8024, 48.6202)
  line L4083 (-27.8024, 48.6202) -> (-27.6119, 48.6202)
  line L4084 (-27.6119, 48.6202) -> (-27.5973, 48.6187)
  line L4085 (-27.8532, 48.4359) -> (-27.9251, 48.364)
  line L4086 (-27.9251, 48.364) -> (-27.9655, 48.2026)
  line L4087 (-27.9655, 48.2026) -> (-27.9655, 47.8877)
  line L4088 (-27.9655, 47.8877) -> (-27.9251, 47.7264)
  line L4089 (-27.9251, 47.7264) -> (-27.8532, 47.6544)
  line L4090 (-27.8532, 47.6544) -> (-27.7847, 47.6202)
  line L4091 (-27.7847, 47.6202) -> (-27.6296, 47.6202)
  line L4092 (-27.6296, 47.6202) -> (-27.5611, 47.6544)
  line L4093 (-27.5611, 47.6544) -> (-27.4892, 47.7264)
  line L4094 (-27.4892, 47.7264) -> (-27.4488, 47.8877)
  line L4095 (-27.4488, 47.8877) -> (-27.4488, 48.2026)
  line L4096 (-27.4488, 48.2026) -> (-27.4892, 48.364)
  line L4097 (-27.4892, 48.364) -> (-27.5611, 48.4359)
  line L4098 (-27.5611, 48.4359) -> (-27.6296, 48.4702)
  line L4099 (-27.6296, 48.4702) -> (-27.7847, 48.4702)
  line L4100 (-27.7847, 48.4702) -> (-27.8532, 48.4359)
  line L4101 (-25.938, 48.6187) -> (-25.9306, 48.6187)
  line L4102 (-25.9306, 48.6187) -> (-25.9238, 48.6159)
  line L4103 (-25.9238, 48.6159) -> (-25.9166, 48.6145)
  line L4104 (-25.9166, 48.6145) -> (-25.9104, 48.6104)
  line L4105 (-25.9104, 48.6104) -> (-25.9036, 48.6075)
  line L4106 (-25.9036, 48.6075) -> (-25.8984, 48.6023)
  line L4107 (-25.8984, 48.6023) -> (-25.8923, 48.5983)
  line L4108 (-25.8923, 48.5983) -> (-25.8881, 48.5921)
  line L4109 (-25.8881, 48.5921) -> (-25.8829, 48.5868)
  line L4110 (-25.8829, 48.5868) -> (-25.8801, 48.5801)
  line L4111 (-25.8801, 48.5801) -> (-25.876, 48.574)
  line L4112 (-25.876, 48.574) -> (-25.8745, 48.5667)
  line L4113 (-25.8745, 48.5667) -> (-25.8717, 48.5598)
  line L4114 (-25.8717, 48.5598) -> (-25.8703, 48.5453)
  line L4115 (-25.8703, 48.5453) -> (-25.8702, 48.5453)
  line L4116 (-25.8702, 48.5453) -> (-25.8702, 48.5452)
  line L4117 (-25.8702, 48.5452) -> (-25.8702, 48.5452)
  line L4118 (-25.8702, 48.5452) -> (-25.8702, 47.6202)
  line L4119 (-25.8702, 47.6202) -> (-25.6595, 47.6202)
  line L4120 (-25.6595, 47.6202) -> (-25.6449, 47.6187)
  line L4121 (-25.6449, 47.6187) -> (-25.6179, 47.6075)
  line L4122 (-25.6179, 47.6075) -> (-25.5972, 47.5868)
  line L4123 (-25.5972, 47.5868) -> (-25.586, 47.5598)
  line L4124 (-25.586, 47.5598) -> (-25.586, 47.5305)
  line L4125 (-25.586, 47.5305) -> (-25.5972, 47.5035)
  line L4126 (-25.5972, 47.5035) -> (-25.6179, 47.4828)
  line L4127 (-25.6179, 47.4828) -> (-25.6449, 47.4716)
  line L4128 (-25.6449, 47.4716) -> (-25.6595, 47.4702)
  line L4129 (-25.6595, 47.4702) -> (-26.231, 47.4702)
  line L4130 (-26.231, 47.4702) -> (-26.2456, 47.4716)
  line L4131 (-26.2456, 47.4716) -> (-26.2726, 47.4828)
  line L4132 (-26.2726, 47.4828) -> (-26.2933, 47.5035)
  line L4133 (-26.2933, 47.5035) -> (-26.3045, 47.5305)
  line L4134 (-26.3045, 47.5305) -> (-26.3045, 47.5598)
  line L4135 (-26.3045, 47.5598) -> (-26.2933, 47.5868)
  line L4136 (-26.2933, 47.5868) -> (-26.2726, 47.6075)
  line L4137 (-26.2726, 47.6075) -> (-26.2456, 47.6187)
  line L4138 (-26.2456, 47.6187) -> (-26.231, 47.6202)
  line L4139 (-26.231, 47.6202) -> (-26.0202, 47.6202)
  line L4140 (-26.0202, 47.6202) -> (-26.0202, 48.3165)
  line L4141 (-26.0202, 48.3165) -> (-26.0827, 48.2541)
  line L4142 (-26.0827, 48.2541) -> (-26.0884, 48.2493)
  line L4143 (-26.0884, 48.2493) -> (-26.0897, 48.2478)
  line L4144 (-26.0897, 48.2478) -> (-26.092, 48.2464)
  line L4145 (-26.092, 48.2464) -> (-26.094, 48.2447)
  line L4146 (-26.094, 48.2447) -> (-26.0959, 48.244)
  line L4147 (-26.0959, 48.244) -> (-26.1022, 48.24)
  line L4148 (-26.1022, 48.24) -> (-26.1974, 48.1924)
  line L4149 (-26.1974, 48.1924) -> (-26.2111, 48.1871)
  line L4150 (-26.2111, 48.1871) -> (-26.2403, 48.1851)
  line L4151 (-26.2403, 48.1851) -> (-26.2681, 48.1943)
  line L4152 (-26.2681, 48.1943) -> (-26.2902, 48.2135)
  line L4153 (-26.2902, 48.2135) -> (-26.3033, 48.2397)
  line L4154 (-26.3033, 48.2397) -> (-26.3054, 48.2688)
  line L4155 (-26.3054, 48.2688) -> (-26.2961, 48.2966)
  line L4156 (-26.2961, 48.2966) -> (-26.2769, 48.3187)
  line L4157 (-26.2769, 48.3187) -> (-26.2645, 48.3265)
  line L4158 (-26.2645, 48.3265) -> (-26.1801, 48.3687)
  line L4159 (-26.1801, 48.3687) -> (-26.0988, 48.4501)
  line L4160 (-26.0988, 48.4501) -> (-26.0076, 48.5868)
  line L4161 (-26.0076, 48.5868) -> (-26.0076, 48.5868)
  line L4162 (-26.0076, 48.5868) -> (-26.0076, 48.5868)
  line L4163 (-26.0076, 48.5868) -> (-26.0075, 48.5869)
  line L4164 (-26.0075, 48.5869) -> (-25.9983, 48.5982)
  line L4165 (-25.9983, 48.5982) -> (-25.9922, 48.6023)
  line L4166 (-25.9922, 48.6023) -> (-25.9869, 48.6075)
  line L4167 (-25.9869, 48.6075) -> (-25.9801, 48.6104)
  line L4168 (-25.9801, 48.6104) -> (-25.974, 48.6144)
  line L4169 (-25.974, 48.6144) -> (-25.9667, 48.6159)
  line L4170 (-25.9667, 48.6159) -> (-25.9599, 48.6187)
  line L4171 (-25.9599, 48.6187) -> (-25.9525, 48.6187)
  line L4172 (-25.9525, 48.6187) -> (-25.9453, 48.6202)
  line L4173 (-25.9453, 48.6202) -> (-25.938, 48.6187)
  line L4174 (-28.5973, 48.6187) -> (-28.5948, 48.6177)
  line L4175 (-28.5948, 48.6177) -> (-28.5921, 48.6175)
  line L4176 (-28.5921, 48.6175) -> (-28.5784, 48.6123)
  line L4177 (-28.5784, 48.6123) -> (-28.4831, 48.5646)
  line L4178 (-28.4831, 48.5646) -> (-28.4768, 48.5607)
  line L4179 (-28.4768, 48.5607) -> (-28.475, 48.5599)
  line L4180 (-28.475, 48.5599) -> (-28.4729, 48.5582)
  line L4181 (-28.4729, 48.5582) -> (-28.4707, 48.5568)
  line L4182 (-28.4707, 48.5568) -> (-28.4694, 48.5553)
  line L4183 (-28.4694, 48.5553) -> (-28.4636, 48.5506)
  line L4184 (-28.4636, 48.5506) -> (-28.416, 48.503)
  line L4185 (-28.416, 48.503) -> (-28.4113, 48.4972)
  line L4186 (-28.4113, 48.4972) -> (-28.4098, 48.4959)
  line L4187 (-28.4098, 48.4959) -> (-28.4084, 48.4937)
  line L4188 (-28.4084, 48.4937) -> (-28.4067, 48.4916)
  line L4189 (-28.4067, 48.4916) -> (-28.4059, 48.4898)
  line L4190 (-28.4059, 48.4898) -> (-28.402, 48.4835)
  line L4191 (-28.402, 48.4835) -> (-28.3543, 48.3882)
  line L4192 (-28.3543, 48.3882) -> (-28.3491, 48.3745)
  line L4193 (-28.3491, 48.3745) -> (-28.3489, 48.3718)
  line L4194 (-28.3489, 48.3718) -> (-28.3479, 48.3693)
  line L4195 (-28.3479, 48.3693) -> (-28.3464, 48.3547)
  line L4196 (-28.3464, 48.3547) -> (-28.3464, 48.2118)
  line L4197 (-28.3464, 48.2118) -> (-28.3479, 48.1972)
  line L4198 (-28.3479, 48.1972) -> (-28.3489, 48.1947)
  line L4199 (-28.3489, 48.1947) -> (-28.3491, 48.192)
  line L4200 (-28.3491, 48.192) -> (-28.3543, 48.1783)
  line L4201 (-28.3543, 48.1783) -> (-28.402, 48.0831)
  line L4202 (-28.402, 48.0831) -> (-28.4059, 48.0768)
  line L4203 (-28.4059, 48.0768) -> (-28.4067, 48.0749)
  line L4204 (-28.4067, 48.0749) -> (-28.4084, 48.0729)
  line L4205 (-28.4084, 48.0729) -> (-28.4098, 48.0706)
  line L4206 (-28.4098, 48.0706) -> (-28.4113, 48.0693)
  line L4207 (-28.4113, 48.0693) -> (-28.416, 48.0636)
  line L4208 (-28.416, 48.0636) -> (-28.4636, 48.016)
  line L4209 (-28.4636, 48.016) -> (-28.4694, 48.0112)
  line L4210 (-28.4694, 48.0112) -> (-28.4707, 48.0097)
  line L4211 (-28.4707, 48.0097) -> (-28.4729, 48.0083)
  line L4212 (-28.4729, 48.0083) -> (-28.475, 48.0066)
  line L4213 (-28.475, 48.0066) -> (-28.4768, 48.0059)
  line L4214 (-28.4768, 48.0059) -> (-28.4831, 48.0019)
  line L4215 (-28.4831, 48.0019) -> (-28.5784, 47.9543)
  line L4216 (-28.5784, 47.9543) -> (-28.5921, 47.949)
  line L4217 (-28.5921, 47.949) -> (-28.5948, 47.9488)
  line L4218 (-28.5948, 47.9488) -> (-28.5973, 47.9478)
  line L4219 (-28.5973, 47.9478) -> (-28.6108, 47.9465)
  line L4220 (-28.6108, 47.9465) -> (-28.36, 47.5882)
  line L4221 (-28.36, 47.5882) -> (-28.3528, 47.5754)
  line L4222 (-28.3528, 47.5754) -> (-28.3464, 47.5468)
  line L4223 (-28.3464, 47.5468) -> (-28.3515, 47.518)
  line L4224 (-28.3515, 47.518) -> (-28.3673, 47.4933)
  line L4225 (-28.3673, 47.4933) -> (-28.3912, 47.4765)
  line L4226 (-28.3912, 47.4765) -> (-28.4198, 47.4702)
  line L4227 (-28.4198, 47.4702) -> (-28.4486, 47.4753)
  line L4228 (-28.4486, 47.4753) -> (-28.4733, 47.491)
  line L4229 (-28.4733, 47.491) -> (-28.4829, 47.5022)
  line L4230 (-28.4829, 47.5022) -> (-28.7938, 47.9464)
  line L4231 (-28.7938, 47.9464) -> (-28.9179, 47.9464)
  line L4232 (-28.9179, 47.9464) -> (-28.9179, 47.5452)
  line L4233 (-28.9179, 47.5452) -> (-28.9193, 47.5305)
  line L4234 (-28.9193, 47.5305) -> (-28.9305, 47.5035)
  line L4235 (-28.9305, 47.5035) -> (-28.9512, 47.4828)
  line L4236 (-28.9512, 47.4828) -> (-28.9782, 47.4716)
  line L4237 (-28.9782, 47.4716) -> (-29.0075, 47.4716)
  line L4238 (-29.0075, 47.4716) -> (-29.0345, 47.4828)
  line L4239 (-29.0345, 47.4828) -> (-29.0552, 47.5035)
  line L4240 (-29.0552, 47.5035) -> (-29.0664, 47.5305)
  line L4241 (-29.0664, 47.5305) -> (-29.0679, 47.5452)
  line L4242 (-29.0679, 47.5452) -> (-29.0679, 48.5452)
  line L4243 (-29.0679, 48.5452) -> (-29.0664, 48.5598)
  line L4244 (-29.0664, 48.5598) -> (-29.0552, 48.5868)
  line L4245 (-29.0552, 48.5868) -> (-29.0345, 48.6075)
  line L4246 (-29.0345, 48.6075) -> (-29.0075, 48.6187)
  line L4247 (-29.0075, 48.6187) -> (-28.9929, 48.6202)
  line L4248 (-28.9929, 48.6202) -> (-28.6119, 48.6202)
  line L4249 (-28.6119, 48.6202) -> (-28.5973, 48.6187)
  line L4250 (-28.9179, 48.0964) -> (-28.6296, 48.0964)
  line L4251 (-28.6296, 48.0964) -> (-28.5611, 48.1306)
  line L4252 (-28.5611, 48.1306) -> (-28.5307, 48.161)
  line L4253 (-28.5307, 48.161) -> (-28.4964, 48.2296)
  line L4254 (-28.4964, 48.2296) -> (-28.4964, 48.337)
  line L4255 (-28.4964, 48.337) -> (-28.5307, 48.4055)
  line L4256 (-28.5307, 48.4055) -> (-28.5611, 48.4359)
  line L4257 (-28.5611, 48.4359) -> (-28.6296, 48.4702)
  line L4258 (-28.6296, 48.4702) -> (-28.9179, 48.4702)
  line L4259 (-28.9179, 48.4702) -> (-28.9179, 48.0964)
  line L4260 (-26.502, 48.6187) -> (-26.475, 48.6075)
  line L4261 (-26.475, 48.6075) -> (-26.4543, 48.5868)
  line L4262 (-26.4543, 48.5868) -> (-26.4431, 48.5598)
  line L4263 (-26.4431, 48.5598) -> (-26.4431, 48.5305)
  line L4264 (-26.4431, 48.5305) -> (-26.4543, 48.5035)
  line L4265 (-26.4543, 48.5035) -> (-26.475, 48.4828)
  line L4266 (-26.475, 48.4828) -> (-26.502, 48.4716)
  line L4267 (-26.502, 48.4716) -> (-26.5167, 48.4702)
  line L4268 (-26.5167, 48.4702) -> (-26.7274, 48.4702)
  line L4269 (-26.7274, 48.4702) -> (-26.7274, 47.5452)
  line L4270 (-26.7274, 47.5452) -> (-26.7288, 47.5305)
  line L4271 (-26.7288, 47.5305) -> (-26.74, 47.5035)
  line L4272 (-26.74, 47.5035) -> (-26.7607, 47.4828)
  line L4273 (-26.7607, 47.4828) -> (-26.7877, 47.4716)
  line L4274 (-26.7877, 47.4716) -> (-26.817, 47.4716)
  line L4275 (-26.817, 47.4716) -> (-26.844, 47.4828)
  line L4276 (-26.844, 47.4828) -> (-26.8647, 47.5035)
  line L4277 (-26.8647, 47.5035) -> (-26.8759, 47.5305)
  line L4278 (-26.8759, 47.5305) -> (-26.8774, 47.5452)
  line L4279 (-26.8774, 47.5452) -> (-26.8774, 48.4702)
  line L4280 (-26.8774, 48.4702) -> (-27.0881, 48.4702)
  line L4281 (-27.0881, 48.4702) -> (-27.1027, 48.4716)
  line L4282 (-27.1027, 48.4716) -> (-27.1298, 48.4828)
  line L4283 (-27.1298, 48.4828) -> (-27.1505, 48.5035)
  line L4284 (-27.1505, 48.5035) -> (-27.1617, 48.5305)
  line L4285 (-27.1617, 48.5305) -> (-27.1617, 48.5598)
  line L4286 (-27.1617, 48.5598) -> (-27.1505, 48.5868)
  line L4287 (-27.1505, 48.5868) -> (-27.1298, 48.6075)
  line L4288 (-27.1298, 48.6075) -> (-27.1027, 48.6187)
  line L4289 (-27.1027, 48.6187) -> (-27.0881, 48.6202)
  line L4290 (-27.0881, 48.6202) -> (-26.5167, 48.6202)
  line L4291 (-26.5167, 48.6202) -> (-26.502, 48.6187)